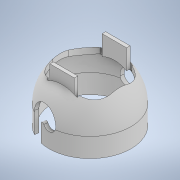
# Autodesk Inventor part: 77. Колпак верхней крышки
Saved by Autodesk Inventor 2021 (Build 250183000, 183)
## iProperties
Created: 2021-03-31
Part Number: 77. Колпак верхней крышки
Material: Типовые
Document SubType Name: Modeling
Designer: Данил
Density: 1 g/cm^3
Appearance: По умолчанию
Author: Данил
Autodesk Inventor part; units mm, degrees
ref_plane "YZ Plane" through (0, 0, 0) normal (1, 0, 0) x (0, 1, 0)
ref_plane "XY Plane" through (0, 0, 0) normal (0, 0, 1) x (1, 0, 0)
sketch "Эскиз1" plane through (0, 0, 0) normal (0, 0, 1) x (1, 0, 0)
  line L0 (0, 17.5) -> (0, -17.5)
  line L1 (23.5, -17.5) -> (23.5, -6.5)
  arc A0 (23.5, -6.5) -> (0, 17) centre (0, -6.5) ccw
  arc A1 (21.5, -6.5) -> (0, 15) centre (0, -6.5) ccw
  line L2 (21.5, -6.5) -> (21.5, -17.5)
  line L3 (21.5, -17.5) -> (23.5, -17.5)
  point P0 (0, 0)
  point P1 (0, 0)
  point P2 (0, 15)
  dimension "d0" = 35
  dimension "d1" = 23.5
  dimension "d2" = 11
  dimension "d3" = 2
  constraints: 8 end point, 4 point on circle, 2 centre point, 2 point on line, 2 vertical, 1 coincident, 1 horizontal, 1 horizontal alignment, 1 midpoint, 1 tangent, 1 other
  measures "d0" distance of L0.start L0.end
  measures "d1" radius of A0
  measures "d2" distance of A0.centre L0.end
  measures "d3" radial gap between concentric circles of A0 A1
revolve "Вращение1" add sketch "Эскиз1" angle 360 about axis through (0, 17.5, 0) along (0, -1, 0)
sketch "Эскиз2" plane through (0, 0, 0) normal (0, 1, 0) x (-1, 0, 0)
  circle A0 centre (0, 0) radius 23.5 projected
  circle A1 centre (0, 0) radius 23.5 projected
  line L0 (0, -23.5) -> (0, 23.5) construction
  line L1 (-4.0807, -23.143) -> (4.0807, 23.143) construction
  point P0 (0, 0)
  point P1 (0, 0)
  dimension "d5" = 10
  constraints: 4 end point, 3 point on circle, 2 midpoint, 1 vertical, 1 vertical alignment
  measures "d5" angle of L0 L1
ref_plane "РабПлоскость1" through (-4.0807, 0, 23.143) normal (-0.1736482, 0, 0.9848078) x (0, -1, 0)
sketch "Эскиз3" plane through (-4.0807, 0, 23.143) normal (-0.1736482, 0, 0.9848078) x (0, -1, 0)
  line L0 (17.5, -23.5) -> (17.5, 23.5) projected
  line L1 (17.5, -21.5) -> (17.5, 21.5) projected
  line L2 (17.5, -7.5) -> (5.4384, -7.5)
  line L3 (17.5, -1) -> (7.5, -1)
  arc A0 (5.4384, 7.5) -> (5.4384, -7.5) centre (5.4384, 0) ccw
  arc A1 (7.0419, 0.8889) -> (5.4384, 7.5) centre (5.4384, 4) ccw
  arc A2 (7.0419, 0.8889) -> (7.5, -1) centre (7.5, 0) ccw
  point P0 (0, 0)
  point P1 (-2.0616, 0)
  point P2 (17.5, -7.5)
  point P3 (17.5, -1)
  dimension "d6" = 6.5
  dimension "d7" = 7.5
  dimension "d8" = 3.5
  dimension "d9" = 1
  dimension "d10" = 10
  constraints: 7 point on circle, 4 end point, 4 tangent, 3 centre point, 2 horizontal, 2 horizontal alignment, 2 point on line
  measures "d6" distance between parallel lines of L2 L3
  measures "d7" radius of A0
  measures "d8" radius of A1
  measures "d9" radius of A2
  measures "d10" distance from line of L0 A2.centre
extrude "Выдавливание1" cut sketch "Эскиз3" against normal up to next
pattern_circular "Круговой массив1" count 2 over 360 about axis through (0, -12, 0) along (0, -1, 0) of "Выдавливание1"
ref_plane "РабПлоскость2" through (0, 20, 0) normal (0, 1, 0) x (-1, 0, 0)
sketch "Эскиз5" plane through (0, 20, 0) normal (0, 1, 0) x (-1, 0, 0)
  arc A0 (-17, -4.417) -> (-9, -15) centre (-6, -4.417) ccw
  arc A1 (-9, -15) -> (-8, -16) centre (-8, -15) ccw
  line L0 (-8, -16) -> (0, -16)
  line L1 (-17, -4.417) -> (-17, 0)
  line L2 (0, -16) -> (0, 0)
  line L3 (0, 0) -> (-17, 0)
  dimension "d17" = 11
  dimension "d19" = 1
  dimension "d20" = 16
  dimension "d21" = 15
  dimension "d22" = 17
  dimension "d23" = 9
  constraints: 8 end point, 4 point on circle, 2 centre point, 2 tangent, 2 vertical, 1 horizontal, 1 horizontal alignment, 1 perpendicular, 1 vertical alignment
  measures "d17" radius of A0
  measures "d19" radius of A1
  measures "d20" distance from line of L2.end L0
  measures "d21" vertical distance of L2.end A0.end
  measures "d22" distance from line of L2.end L1
  measures "d23" horizontal distance of L0.end A0.end
extrude "Выдавливание2" cut sketch "Эскиз5" against normal through all both and the other way through all
mirror "Зеркальное отражение1" about plane through (0, 0, 0) normal (1, 0, 0) of "Выдавливание2"
mirror "Зеркальное отражение2" about plane through (0, 0, 0) normal (0, 0, 1) of "Выдавливание2", "Зеркальное отражение1"
sketch "Эскиз6" plane through (8, 5.4269, -16) normal (0, 0, 1) x (1, 0, 0)
  arc A0 (0, 0) -> (-16, 0) centre (-8, -11.9269) ccw projected
  arc A1 (0, 3.3129) -> (-16, 3.3129) centre (-8, -11.9269) ccw projected
  line L0 (-15, 0.6131) -> (-15, 12.0731)
  line L1 (-15, 12.0731) -> (-1, 12.0731)
  line L2 (-1, 12.0731) -> (-1, 0.6131)
  line L3 (-29.5, -22.9269) -> (-3.2858, -22.9269) projected
  point P0 (-8, -5.4269)
  point P1 (-8, 12.0731)
  point P2 (-18.885, -22.9269)
  dimension "d26" = 14
  dimension "d27" = 35
  constraints: 6 end point, 2 perpendicular, 2 point on circle, 1 horizontal alignment, 1 midpoint, 1 vertical, 1 vertical alignment
  measures "d26" distance of L0.end L1.end
  measures "d27" distance between parallel lines of L3 L1
extrude "Выдавливание3" add sketch "Эскиз6" along normal blind 2
mirror "Зеркальное отражение3" about plane through (0, 0, 0) normal (0, 0, 1) of "Выдавливание3"
